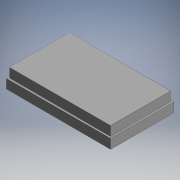
# Autodesk Inventor part: ManifoldLid0
Saved by Autodesk Inventor 2018 (Build 220112000, 112)
## iProperties
Created: 2018-10-10
Part Number: ManifoldLid0
Material: Generic
Document SubType Name: Modeling
Designer: Isaac Newcomb
Density: 1 g/cm^3
Appearance: Default
Author: Isaac Newcomb
Autodesk Inventor part; units mm, degrees
ref_plane "YZ Plane" through (0, 0, 0) normal (1, 0, 0) x (0, 1, 0)
ref_plane "XZ Plane" through (0, 0, 0) normal (0, 1, 0) x (-1, 0, 0)
ref_plane "XY Plane" through (0, 0, 0) normal (0, 0, 1) x (1, 0, 0)
sketch "Base Sketch" plane through (0, 0, 0) normal (0, 1, 0) x (-1, 0, 0)
  line L0 (0, 0) -> (-33, 0)
  line L1 (-33, 0) -> (-33, -20)
  line L2 (-33, -20) -> (0, -20)
  line L3 (0, -20) -> (0, 0)
  dimension "d0" = 33
  dimension "d1" = 20
  constraints: 8 end point, 2 parallel, 1 horizontal, 1 perpendicular
  measures "d0" distance of L2.end L1.end
  measures "d1" distance of L2.end L0.start
extrude "Base" add sketch "Base Sketch" along normal blind 3
sketch "Inner Part Sketch" plane through (0, 3, 0) normal (0, -1, 0) x (1, 0, 0)
  line L0 (0, 0) -> (33, 0) construction
  line L1 (33, 0) -> (33, -20) construction
  line L2 (33, -20) -> (0, -20) construction
  line L3 (0, -20) -> (0, 0) construction
  line L4 (0.5, -19.5) -> (32.5, -19.5)
  line L5 (32.5, -19.5) -> (32.5, -0.5)
  line L6 (32.5, -0.5) -> (0.5, -0.5)
  line L7 (0.5, -0.5) -> (0.5, -19.5)
  dimension "d4" = 0.5
  constraints: 8 end point, 3 other
  measures "d4" distance between parallel lines of L2 L4
extrude "Inner Part" add sketch "Inner Part Sketch" against normal blind 3
equation "\"d0\" = ManifoldInnerWidth + 2 * ManifoldWallThickness"
equation "\"d1\" = ManifoldOuterDepth"
equation "\"d4\" = ManifoldWallThickness"
equation "\"ManifoldInnerWidth\" = 32"
equation "\"ManifoldWallThickness\" = 0.5"
equation "\"ManifoldOuterDepth\" = 20"
body "Solid1"
